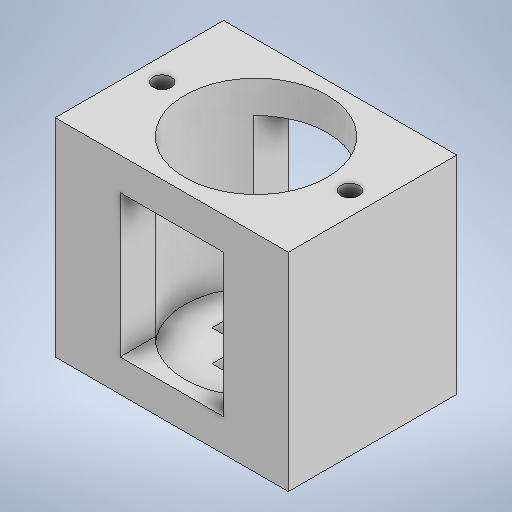
# Autodesk Inventor part: Motorblock_N20
Saved by Autodesk Inventor 2025 (Build 290162000, 162)
## iProperties
Created: 2026-07-13
Part Number: Motorblock_N20
Material: Generisch
Document SubType Name: Modeling
Designer: wavid
Mass: 16.5968 g
Surface Area: 76.2472 cm^2
Volume: 16.5968 cm^3
Density: 1 g/cm^3
Appearance: Vorgabe
Author: wavid
Autodesk Inventor part; units mm, degrees
ref_plane "YZ Plane" through (0, 0, 0) normal (1, 0, 0) x (0, 1, 0)
ref_plane "XZ Plane" through (0, 0, 0) normal (0, 1, 0) x (-1, 0, 0)
sketch "Skizze1" plane through (0, 0, 0) normal (0, 0, 1) x (1, 0, 0)
  line L0 (-18, -13) -> (18, -13)
  line L1 (18, -13) -> (18, 13)
  line L2 (18, 13) -> (-18, 13)
  line L3 (-18, 13) -> (-18, -13)
  constraints: 8 end point, 2 parallel, 1 horizontal, 1 perpendicular
extrude "Extrusion1" add sketch "Skizze1" along normal blind 32
sketch "Skizze2" plane through (0, 0, 0) normal (0, 0, 1) x (1, 0, 0)
  circle A0 centre (0, 0) radius 2.5
  constraints: 1 centre point
extrude "Extrusion2" cut sketch "Skizze2" along normal blind 4.2
sketch "Skizze3" plane through (0, 0, 0) normal (0, 0, 1) x (1, 0, 0)
  line L0 (3.3, -1) -> (5.8, -1)
  line L1 (5.8, -1) -> (5.8, 1)
  line L2 (5.8, 1) -> (3.3, 1)
  line L3 (3.3, 1) -> (3.3, -1)
  constraints: 8 end point, 2 parallel, 1 horizontal, 1 perpendicular
extrude "Extrusion3" cut sketch "Skizze3" along normal blind 4.2
sketch "Skizze4" plane through (0, 0, 0) normal (0, 0, 1) x (1, 0, 0)
  line L0 (-5.8, -1) -> (-3.3, -1)
  line L1 (-3.3, -1) -> (-3.3, 1)
  line L2 (-3.3, 1) -> (-5.8, 1)
  line L3 (-5.8, 1) -> (-5.8, -1)
  constraints: 8 end point, 2 parallel, 1 horizontal, 1 perpendicular
extrude "Extrusion4" cut sketch "Skizze4" along normal blind 4.2
sketch "Skizze5" plane through (0, 0, 0) normal (0, 0, 1) x (1, 0, 0)
  line L0 (-1, 3.3) -> (1, 3.3)
  line L1 (1, 3.3) -> (1, 5.8)
  line L2 (1, 5.8) -> (-1, 5.8)
  line L3 (-1, 5.8) -> (-1, 3.3)
  constraints: 8 end point, 2 parallel, 1 horizontal, 1 perpendicular
extrude "Extrusion5" cut sketch "Skizze5" along normal blind 4.2
sketch "Skizze6" plane through (0, 0, 0) normal (0, 0, 1) x (1, 0, 0)
  line L0 (-1, -5.8) -> (1, -5.8)
  line L1 (1, -5.8) -> (1, -3.3)
  line L2 (1, -3.3) -> (-1, -3.3)
  line L3 (-1, -3.3) -> (-1, -5.8)
  constraints: 8 end point, 2 parallel, 1 horizontal, 1 perpendicular
extrude "Extrusion6" cut sketch "Skizze6" along normal blind 4.2
sketch "Skizze7" plane through (0, 0, 0) normal (0, 0, 1) x (1, 0, 0)
  circle A0 centre (-14.5, 0) radius 1.4
  constraints: 1 centre point
extrude "Extrusion7" cut sketch "Skizze7" along normal blind 32.2
sketch "Skizze8" plane through (0, 0, 0) normal (0, 0, 1) x (1, 0, 0)
  circle A0 centre (14.5, 0) radius 1.4
  constraints: 1 centre point
extrude "Extrusion8" cut sketch "Skizze8" along normal blind 32.2
ref_plane "Arbeitsebene1" through (0, 0, 32) normal (0, 0, 1) x (1, 0, 0)
sketch "Skizze9" plane through (0, 0, 32) normal (0, 0, 1) x (1, 0, 0)
  circle A0 centre (0, 0) radius 11
  constraints: 1 centre point
extrude "Extrusion9" cut sketch "Skizze9" against normal blind 28
sketch "Skizze10" plane through (0, 0, 0) normal (0, 1, 0) x (-1, 0, 0)
  line L0 (-8, 5) -> (8, 5)
  line L1 (8, 5) -> (8, 27)
  line L2 (8, 27) -> (-8, 27)
  line L3 (-8, 27) -> (-8, 5)
  constraints: 8 end point, 2 parallel, 1 horizontal, 1 perpendicular
extrude "Extrusion10" cut sketch "Skizze10" along normal mid plane 30
